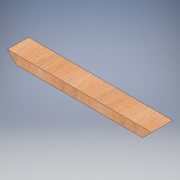
# Autodesk Inventor part: Short Wall 45 Diagonal Piece
Saved by Autodesk Inventor 2016 (Build 200138000, 138)
## iProperties
Created: 2015-07-05
Part Number: Short Wall 45 Diagonal Piece
Material: Wood (Birch)
Document SubType Name: Modeling
Designer: steele
Density: 0.55 g/cm^3
Appearance: Birch - Natural Polished
Author: steele
Autodesk Inventor part; units mm, degrees
ref_plane "YZ Plane" through (0, 0, 0) normal (1, 0, 0) x (0, 1, 0)
ref_plane "XZ Plane" through (0, 0, 0) normal (0, 1, 0) x (-1, 0, 0)
ref_plane "XY Plane" through (0, 0, 0) normal (0, 0, 1) x (1, 0, 0)
sketch "Sketch2" plane through (0, 0, 0) normal (0, 0, 1) x (1, 0, 0)
  line L0 (-276.0165, -21.3406) -> (257.3835, -21.3406)
  line L1 (295.4835, 16.7594) -> (-314.1165, 16.7594)
  line L2 (-285.4373, -16.1896) -> (295.4835, 16.7594) construction
  line L3 (266.9116, -14.2408) -> (-314.1165, 16.7594) construction
  line L4 (-314.1165, 16.7594) -> (-276.0165, -21.3406)
  line L5 (-314.1165, 16.7594) -> (-260.2349, 16.7594) construction
  line L6 (295.4835, 16.7594) -> (257.3835, -21.3406)
  line L7 (295.4835, 16.7594) -> (349.3651, 16.7594) construction
  point P0 (0, 0)
  dimension "d10" = 45
  dimension "d11" = 135
  dimension "d14" = 609.6
  dimension "d15" = 38.1
  constraints: 16 end point, 3 horizontal, 2 equal length, 2 point on line, 1 parallel
  measures "d10" angle of L4 L5
  measures "d11" angle of L6 L7
  measures "d14" distance of L1.start L1.end
  measures "d15" distance between parallel lines of L0 L1
extrude "Extrusion2" add sketch "Sketch2" along normal mid plane 88.9
body "Solid2"
